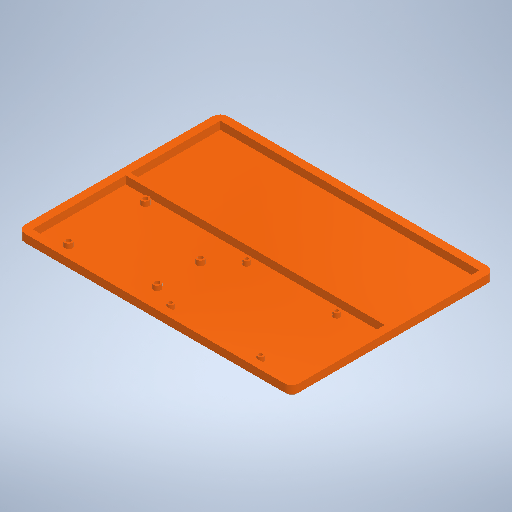
# Autodesk Inventor part: Electronic Base
Saved by Autodesk Inventor 2025.2 (Build 292293000, 293)
## iProperties
Created: 2025-02-05
Part Number: Electronic Base
Material: Generic
Document SubType Name: Modeling
Designer: caomi
Density: 1 g/cm^3
Appearance: Default
Author: caomi
Autodesk Inventor part; units mm, degrees
ref_plane "YZ Plane" through (0, 0, 0) normal (1, 0, 0) x (0, 1, 0)
ref_plane "XZ Plane" through (0, 0, 0) normal (0, 1, 0) x (-1, 0, 0)
ref_plane "XY Plane" through (0, 0, 0) normal (0, 0, 1) x (1, 0, 0)
sketch "Sketch1" plane through (0, 0, 0) normal (0, 1, 0) x (-1, 0, 0)
  line L0 (88.5, 65.5) -> (-88.5, 65.5)
  line L1 (-88.5, 65.5) -> (-88.5, -65.5)
  line L2 (-88.5, -65.5) -> (88.5, -65.5)
  line L3 (88.5, -65.5) -> (88.5, 65.5)
  line L4 (88.5, 65.5) -> (-88.5, -65.5) construction
  line L5 (-88.5, 65.5) -> (88.5, -65.5) construction
  line L6 (83.5, -60.5) -> (-83.5, -60.5)
  line L7 (-83.5, -60.5) -> (-83.5, -2.5)
  line L8 (-83.5, -2.5) -> (83.5, -2.5)
  line L9 (83.5, -2.5) -> (83.5, -60.5)
  line L10 (83.5, -60.5) -> (-83.5, -2.5) construction
  line L11 (-83.5, -60.5) -> (83.5, -2.5) construction
  circle A0 centre (66.26, 5.04) radius 1.5
  circle A1 centre (67.53, 53.3) radius 1.5
  circle A2 centre (15.46, 20.28) radius 1.5
  circle A3 centre (15.46, 48.22) radius 1.5
  line L12 (81.5, 2.5) -> (13.5, 2.5) construction
  line L13 (13.5, 2.5) -> (13.5, 55.84) construction
  line L14 (13.5, 55.84) -> (81.5, 55.84) construction
  line L15 (81.5, 55.84) -> (81.5, 2.5) construction
  line L16 (3.5, 2.5) -> (-81.5, 2.5) construction
  line L17 (-81.5, 2.5) -> (-81.5, 58.5) construction
  line L18 (-81.5, 58.5) -> (3.5, 58.5) construction
  line L19 (3.5, 58.5) -> (3.5, 2.5) construction
  circle A4 centre (0, 6) radius 1.1
  circle A5 centre (0, 55) radius 1.1
  circle A6 centre (-58, 6) radius 1.1
  circle A7 centre (-58, 55) radius 1.1
  line L20 (0, 0) -> (-136.9444, 0) construction
  line L21 (0, 0) -> (0, -40.8719) construction
  line L22 (9.5, 0.5) -> (83.5, 0.5)
  line L23 (83.5, 0.5) -> (83.5, 57.84)
  line L24 (-83.5, 0.5) -> (7.5, 0.5)
  line L25 (7.5, 60.5) -> (-83.5, 60.5)
  line L26 (-83.5, 60.5) -> (-83.5, 0.5)
  circle A8 centre (66.26, 5.04) radius 2.5
  circle A9 centre (67.53, 53.3) radius 2.5
  circle A10 centre (15.46, 20.28) radius 2.5
  circle A11 centre (15.46, 48.22) radius 2.5
  circle A12 centre (0, 6) radius 2.1
  circle A13 centre (0, 55) radius 2.1
  circle A14 centre (-58, 6) radius 2.1
  circle A15 centre (-58, 55) radius 2.1
  line L27 (9.5, 0.5) -> (7.5, 0.5)
  line L28 (7.5, 60.5) -> (83.5, 60.5)
  line L29 (83.5, 60.5) -> (83.5, 57.84)
  point P0 (0, -31.5)
  point P1 (13.5, 21.8319)
  point P2 (13.5, 18.7281)
  point P3 (13.5, 49.7719)
  point P4 (13.5, 46.6681)
  dimension "d0" = 167
  dimension "d1" = 58
  dimension "d2" = 3
  dimension "d3" = 50.8
  dimension "d4" = 15.24
  dimension "d5" = 17.78
  dimension "d6" = 45.72
  dimension "d7" = 66.04
  dimension "d8" = 85
  dimension "d9" = 56
  dimension "d10" = 2.2
  dimension "d11" = 3.5
  dimension "d12" = 3.5
  dimension "d13" = 3.5
  dimension "d15" = 2
  dimension "d16" = 5
  dimension "d23" = 68
  dimension "d24" = 53.34
  dimension "d25" = 13.97
  dimension "d26" = 2.54
  dimension "d27" = 2
  dimension "d28" = 2
  dimension "d29" = 1
  dimension "d30" = 1
  dimension "d31" = 1
  dimension "d32" = 1
  dimension "d33" = 1
  dimension "d34" = 1
  dimension "d35" = 1
  dimension "d36" = 1
  dimension "d40" = 5
  dimension "d41" = 5
  dimension "d42" = 5
  dimension "d43" = 2
  dimension "d44" = 58
  constraints: 60 end point, 16 centre point, 10 parallel, 6 equal radius, 6 perpendicular, 5 horizontal, 4 midpoint, 3 vertical alignment, 2 collinear, 2 horizontal alignment, 1 vertical, 3 other
  measures "d0" distance of L6.start L6.end
  measures "d1" distance of L6.end L7.end
  measures "d2" diameter of A0
  measures "d3" distance from line of A1.centre L12
  measures "d4" distance from line of A0.centre L15
  measures "d5" distance from line of L12 A2.centre
  measures "d6" distance from line of L12 A3.centre
  measures "d7" distance from line of L15 A3.centre
  measures "d8" distance of L17.end L18.end
  measures "d9" distance of L16.end L17.end
  measures "d10" diameter of A4
  measures "d11" distance from line of L16 A4.centre
  measures "d12" distance from line of A4.centre L19
  measures "d13" distance from line of L18 A5.centre
  measures "d15" distance between parallel lines of L7 L17
  measures "d16" distance between parallel lines of L16 L8
  measures "d23" distance of L13.end L14.end
  measures "d24" distance of L14.end L12.start
  measures "d25" distance from line of L15 A1.centre
  measures "d26" distance from line of L12 A0.centre
  measures "d27" distance between parallel lines of L12 L22
  measures "d28" distance between parallel lines of L16 L24
  measures "d29" radial gap between concentric circles of A0 A8
  measures "d30" radial gap between concentric circles of A1 A9
  measures "d31" radial gap between concentric circles of A2 A10
  measures "d32" radial gap between concentric circles of A3 A11
  measures "d33" radial gap between concentric circles of A4 A12
  measures "d34" radial gap between concentric circles of A5 A13
  measures "d35" radial gap between concentric circles of A6 A14
  measures "d36" radial gap between concentric circles of A7 A15
  measures "d40" distance between parallel lines of L0 L25
  measures "d41" distance between parallel lines of L1 L26
  measures "d42" distance between parallel lines of L2 L6
  measures "d43" distance between parallel lines of L26 L17
  measures "d44" distance of A4.centre A6.centre
extrude "Extrusion1" add sketch "Sketch1" against normal blind 2 contours L3 L2 L1 L0 | L6 L7 L8 L9 | L27 L24 L26 L25 L28 L29 L23 L22 | A8 | A9 | A10 | A11 | A12 | A13 | A14 | A15
extrude "Extrusion2" add sketch "Sketch1" along normal blind 5 contours L3 L2 L1 L0
extrude "Extrusion3" add sketch "Sketch1" along normal blind 3 contours A8 | A9 | A10 | A11 | A12 | A13 | A14 | A15
fillet "Fillet1" radius 5 4 edges at (-88.5, 1.5, -65.5) (88.5, 1.5, -65.5) (88.5, 1.5, 65.5) (-88.5, 1.5, 65.5)
chamfer "Chamfer1" distance 2 angle 45 8 edges at (0, -2, 65.5) (-87.0355, -2, 64.0355) (-88.5, -2, 0) (-87.0355, -2, -64.0355) (0, -2, -65.5) (87.0355, -2, -64.0355) (88.5, -2, 0) (87.0355, -2, 64.0355)
equation "\"d12\" = d11"
equation "\"d13\" = d11"
body "Solid1"
